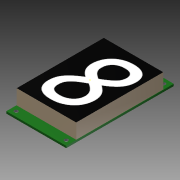
# Autodesk Inventor part: Big7seg
Saved by Autodesk Inventor 2015 (Build 190159000, 159)
## iProperties
Created: 2016-04-26
Part Number: Big7seg
Material: 一般
Document SubType Name: Modeling
Designer: yamashita1
Density: 1 g/cm^3
Appearance: 既定
Author: yamashita1
Autodesk Inventor part; units mm, degrees
ref_plane "YZ Plane" through (0, 0, 0) normal (1, 0, 0) x (0, 1, 0)
ref_plane "XZ Plane" through (0, 0, 0) normal (0, 1, 0) x (-1, 0, 0)
ref_plane "XY Plane" through (0, 0, 0) normal (0, 0, 1) x (1, 0, 0)
sketch "スケッチ1" plane through (0, 0, 0) normal (0, 0, 1) x (1, 0, 0)
  line L0 (-24, 43) -> (24, 43)
  line L1 (24, 43) -> (24, -43)
  line L2 (24, -43) -> (-24, -43)
  line L3 (-24, -43) -> (-24, 43)
  point P0 (0, 0)
  point P1 (0, 43)
  point P2 (24, 0)
  dimension "d0" = 48
  dimension "d1" = 86
  constraints: 8 end point, 2 midpoint, 2 parallel, 1 horizontal, 1 horizontal alignment, 1 perpendicular, 1 vertical alignment
  measures "d0" distance of L1.end L2.end
  measures "d1" distance of L0.end L1.end
extrude "押し出し1" add sketch "スケッチ1" along normal blind 1.6
sketch "スケッチ2" plane through (0, 0, 1.6) normal (0, 0, 1) x (1, 0, 0)
  line L0 (-23.75, 34.8) -> (23.75, 34.8)
  line L1 (23.75, 34.8) -> (23.75, -34.8)
  line L2 (23.75, -34.8) -> (-23.75, -34.8)
  line L3 (-23.75, -34.8) -> (-23.75, 34.8)
  point P0 (0, 0)
  point P1 (0, 34.8)
  point P2 (23.75, 0)
  dimension "d4" = 47.5
  dimension "d5" = 69.6
  constraints: 8 end point, 2 midpoint, 2 parallel, 1 horizontal, 1 horizontal alignment, 1 perpendicular, 1 vertical alignment
  measures "d4" distance of L1.end L2.end
  measures "d5" distance of L0.end L1.end
extrude "押し出し2" add sketch "スケッチ2" along normal blind 12
sketch "スケッチ3" plane through (0, 0, 1.6) normal (0, 0, 1) x (1, 0, 0)
  line L0 (-24, -43) -> (24, -43) projected
  line L1 (-24, 43) -> (-24, -43) projected
  line L2 (24, -43) -> (24, 43) projected
  line L3 (24, 43) -> (-24, 43) projected
  circle A0 centre (-20, -39) radius 1.5
  circle A1 centre (20, -39) radius 1.5
  circle A2 centre (-20, 39) radius 1.5
  circle A3 centre (20, 39) radius 1.5
  point P0 (0, 0)
  dimension "d8" = 4
  dimension "d9" = 4
  dimension "d10" = 4
  dimension "d11" = 4
  dimension "d12" = 3
  constraints: 4 centre point, 4 coincident, 3 equal radius, 2 horizontal alignment, 2 vertical alignment
  measures "d8" distance from line of L0 point (-20, -39)
  measures "d9" distance from line of L1 point (-20, -39)
  measures "d10" distance from line of L2 point (20, -39)
  measures "d11" distance from line of point (-20, 39) L3
  measures "d12" diameter of A0
extrude "押し出し3" cut sketch "スケッチ3" against normal blind 1.6 contours A0 | A1 | A2 | A3
sketch "スケッチ4" plane through (0, 0, 13.6) normal (0, 0, 1) x (1, 0, 0)
  line L0 (-19.4086, 28.472) -> (45.9399, 28.472) construction
  line L1 (45.9399, 28.472) -> (45.9399, -30.0693) construction
  line L2 (45.9399, -30.0693) -> (-19.4086, -30.0693) construction
  line L3 (-19.4086, -30.0693) -> (-19.4086, 28.472) construction
  point P0 (0, 0)
  constraints: 2 other
